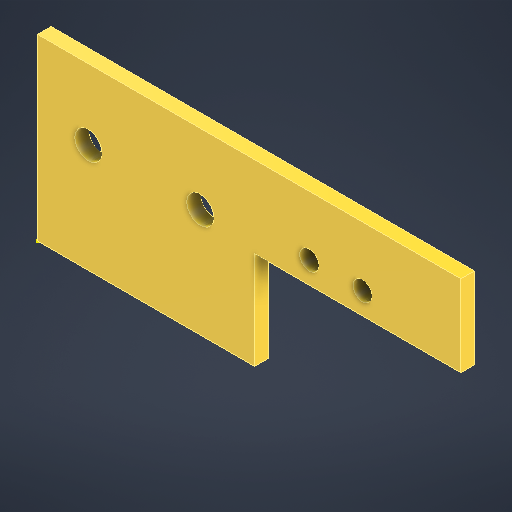
# Autodesk Inventor part: Part1
Saved by Autodesk Inventor 2027.1 (Build 311270010, 270A)
## iProperties
Created: 2026-07-19
Part Number: Part1
Material: Generic
Document SubType Name: Sheet Metal
Designer: MSI
Density: 1 g/cm^3
Sheet Metal Rule: Default_mm
Appearance: Glossy - Gold
Author: MSI
Autodesk Inventor part; units mm, degrees
ref_plane "YZ Plane" through (0, 0, 0) normal (1, 0, 0) x (0, 1, 0)
ref_plane "XZ Plane" through (0, 0, 0) normal (0, 1, 0) x (-1, 0, 0)
ref_plane "XY Plane" through (0, 0, 0) normal (0, 0, 1) x (1, 0, 0)
sketch "Sketch1" plane through (0, 0, 0) normal (0, 0, 1) x (1, 0, 0)
  line L0 (0, 0) -> (0, 33)
  line L1 (0, 33) -> (40, 33)
  line L2 (40, 33) -> (78.0336, 33)
  line L3 (78.0336, 18) -> (40, 18)
  line L4 (40, 18) -> (40, 0)
  line L5 (40, 0) -> (0, 0)
  circle A0 centre (9.3675, 20) radius 2.5
  circle A1 centre (30, 20) radius 2.5
  circle A2 centre (50.0876, 22) radius 1.75
  circle A3 centre (59.8876, 22) radius 1.75
  line L6 (40, 18) -> (55, 18)
  line L7 (78.0336, 18) -> (78.0336, 33)
  point P0 (0, 16.5)
  dimension "d0" = 40
  dimension "d1" = 33
  dimension "d2" = 5
  dimension "d3" = 5
  dimension "d4" = 10
  dimension "d5" = 10
  dimension "d6" = 20
  dimension "d7" = 20
  dimension "d9" = 3.5
  dimension "d10" = 3.5
  dimension "d11" = 9.8
  dimension "d12" = 4
  dimension "d15" = 15
  constraints: 16 end point, 4 centre point, 4 perpendicular, 1 midpoint, 1 point on line, 1 vertical
  measures "d0" distance between parallel lines of L4 L0
  measures "d1" distance between parallel lines of L5 L1
  measures "d2" diameter of A0
  measures "d3" diameter of A1
  measures "d4" distance of point (0, 16.5) A0.centre
  measures "d5" distance from line of L4 A1.centre
  measures "d6" distance from line of L5 A1.centre
  measures "d7" distance from line of L5 A0.centre
  measures "d9" diameter of A2
  measures "d10" diameter of A3
  measures "d11" distance of A3.centre A2.centre
  measures "d12" distance from line of L3 A3.centre
  measures "d15" distance of L3.end L6.end
extrude "Extrusion1" add sketch "Sketch1" along normal blind 2.5
sketch "Sketch3" plane through (0, 0, 2.5) normal (0, 0, 1) x (1, 0, 0)
  point P0 (0, 0)
sketch "Sketch4" plane through (0, 0, 2.5) normal (0, 0, 1) x (1, 0, 0)
  point P0 (0, 0)
equation "\"BendRadius\" = Thickness"
equation "\"BendReliefWidth\" = Thickness"
equation "\"BendReliefDepth\" = 0.5 * Thickness"
equation "\"CornerReliefSize\" = 4 * Thickness"
equation "\"MinimumRemnant\" = 2 * Thickness"
equation "\"TransitionRadius\" = BendRadius"
equation "\"JacobiRadiusSize\" = BendRadius"
equation "\"GapSize\" = Thickness"
equation "\"Thickness\" = 0.5"
body "Solid1"
